Cam Halter Bed (Autodesk Fusion 360 design; units mm, degrees)
Autodesk Fusion 360 part; units mm, degrees
sketch "Sketch1" plane through (0, 0, 0) normal (0, 0, 1) x (1, 0, 0)
  circle A0 centre (0, 0) radius 3.7
  circle A1 centre (0, 0) radius 6
  line L0 (-25, -13.2) -> (25, -13.2)
  line L1 (25, -13.2) -> (25, -17.2)
  line L2 (25, -17.2) -> (-25, -17.2)
  line L3 (-25, -17.2) -> (-25, -13.2)
  line L4 (-6, 0) -> (6, 0)
  line L5 (6, 0) -> (6, -13.2)
  line L6 (6, -13.2) -> (-6, -13.2)
  line L7 (-6, -13.2) -> (-6, 0)
  point P0 (0, -13.2)
  dimension "d1" = 7.4
  dimension "d2" = 12
  dimension "d7" = 50
  dimension "d8" = 13.2
  dimension "d30" = 4
  constraint coincident A0.centre A1.centre
  constraint horizontal L0
  constraint vertical L1
  constraint horizontal L2
  constraint vertical L3
  constraint midpoint L0 P0
  constraint vertical A0.centre P0
  constraint horizontal L4
  constraint vertical L5
  constraint horizontal L6
  constraint vertical L7
  constraint collinear L0 L6
  constraint tangent A1 L7
  constraint tangent A1 L5
  constraint coincident A0.centre L4
  measures "d1" diameter of A0
  measures "d2" diameter of A1
  measures "d7" distance of L0.start L0.end
  measures "d8" distance of A0.centre L0
  measures "d30" distance of L0.start L2.end
extrude "Extrude1" add sketch "Sketch1" along normal blind 2 contours A0 L4 | A0 A1 L4 | A0 A1 L4 | A0 L4
extrude "Extrude2" add sketch "Sketch1" along normal blind 18 contours A0 A1 L4 | A0 A1 L4
extrude "Extrude3" add sketch "Sketch1" along normal blind 12 contours A1 L0 L5 L6 L7
extrude "Extrude9" add 1 faces at (2, -13.2, 8) along direction (0, -1, 0) blind 1
draft "Draft1" angle 35 neutral plane through (-6, -13.2, 0) pull (0, 0, -1) 1 faces at (2, -14.2, 8)
sketch "Sketch5" plane through (0, -9.5283, -6.6718) normal (0, -0.819152, -0.573576) x (1, 0, 0)
  line L0 (-6, 8.1448) -> (6, 8.1448)
  line L1 (6, 8.1448) -> (6, 22.7941)
  line L2 (6, 22.7941) -> (-6, 22.7941)
  line L3 (-6, 22.7941) -> (-6, 8.1448)
  circle A0 centre (0, 22.2702) radius 35
  dimension "d44" = 70
  measures "d44" diameter of A0
extrude "Extrude10" add sketch "Sketch5" along normal blind 1.2 contours L0 L1 L2 L3 | A0
